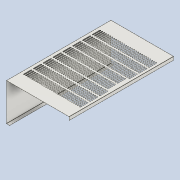
# Autodesk Inventor part: Tapa_superior_sup_ch
Saved by Autodesk Inventor 2021 (Build 250183000, 183)
## iProperties
Created: 2021-05-16
Part Number: Tapa_superior_sup_ch
Material: Acero AISI 1006 85 LC
Document SubType Name: Chapa
Designer: Admin
Density: 7.872 g/cm^3
Sheet Metal Rule: Por defecto_mm
Appearance: Acero
Author: Admin
Autodesk Inventor part; units mm, degrees
(part 1 of 2)
ref_plane "YZ Plane" through (0, 0, 0) normal (1, 0, 0) x (0, 1, 0)
ref_plane "XZ Plane" through (0, 0, 0) normal (0, 1, 0) x (-1, 0, 0)
ref_plane "XY Plane" through (0, 0, 0) normal (0, 0, 1) x (1, 0, 0)
sketch "Boceto1" plane through (0, 0, 0) normal (0, 1, 0) x (-1, 0, 0)
  line L0 (0, 0) -> (383.48, 0)
  line L1 (383.48, 0) -> (383.48, -637.48)
  line L2 (383.48, -637.48) -> (0, -637.48)
  line L3 (0, -637.48) -> (0, 0)
  dimension "d0" = 383.48
  dimension "d1" = 637.48
  measures "d0" distance of L1.end L2.end
  measures "d1" distance of L0.end L1.end
extrude "Placa1" add sketch "Boceto1" along normal blind 0.5
sketch "Boceto2" plane through (-0.5, 0.5, -637.48) normal (1, 0, 0) x (0, -1, 0)
  line L0 (0, 637.48) -> (0, 0)
  line L1 (0, 0) -> (20, 0)
  line L2 (20, 0) -> (20, 637.48)
  line L3 (20, 637.48) -> (0, 637.48)
  constraints: 6 end point, 1 horizontal, 1 perpendicular, 1 vertical
edge flange "Pestaña1" height 20 angle 90 thickness 0.5 bend radius 0.5 thickness toward (1, 0, 0) relief tear relief width 0.5 relief depth 0.25 edges at (0, 0.5, -318.74) wall of the first edge with corners at (-0.5, 0.5, 0) (-0.5, 0.5, -637.48) (-0.5, -19.5, -637.48) (-0.5, -19.5, 0)
bend "Doblez1"
corner "Esquina1"
sketch "Boceto3" plane through (-382.98, 0.5, 0) normal (-1, 0, 0) x (0, 1, 0)
  line L0 (0, -637.48) -> (0, 0)
  line L1 (0, 0) -> (-228.48, 0)
  line L2 (-228.48, 0) -> (-228.48, -637.48)
  line L3 (-228.48, -637.48) -> (0, -637.48)
  constraints: 6 end point, 1 horizontal, 1 perpendicular, 1 vertical
edge flange "Pestaña2" height 228.48 angle 90 thickness 0.5 bend radius 0.5 thickness toward (-1, 0, 0) relief tear relief width 0.5 relief depth 0.25 edges at (-383.48, 0.5, -318.74) wall of the first edge with corners at (-382.98, 0.5, -637.48) (-382.98, 0.5, 0) (-382.98, -227.98, 0) (-382.98, -227.98, -637.48)
bend "Doblez2"
corner "Esquina2"
sketch "Boceto4" plane through (-383.48, -227.48, 0) normal (0, -1, 0) x (-1, 0, 0)
  line L0 (0, -637.48) -> (0, 0)
  line L1 (0, 0) -> (-20, 0)
  line L2 (-20, 0) -> (-20, -637.48)
  line L3 (-20, -637.48) -> (0, -637.48)
  constraints: 6 end point, 1 horizontal, 1 perpendicular, 1 vertical
edge flange "Pestaña3" height 20 angle 90 thickness 0.5 bend radius 0.5 thickness toward (0, -1, 0) relief tear relief width 0.5 relief depth 0.25 edges at (-383.48, -227.98, -318.74) wall of the first edge with corners at (-383.48, -227.48, -637.48) (-383.48, -227.48, 0) (-363.48, -227.48, 0) (-363.48, -227.48, -637.48)
bend "Doblez3"
corner "Esquina3"
sketch "Boceto5" plane through (0, 0.5, 0) normal (0, 1, 0) x (1, 0, 0)
  line L0 (0, 637.48) -> (0, 0) projected
  line L1 (0, 318.74) -> (-382.98, 318.74)
  line L2 (-382.98, 637.48) -> (-382.98, 0) projected
  line L3 (-1, 0) -> (-382.48, 0) projected
  line L4 (-382.48, 637.48) -> (-1, 637.48) projected
  line L5 (-383.48, 0) -> (-383.48, 637.48) projected
  line L6 (0, 0) -> (0, 637.48) projected
  line L7 (-31.95, 313.74) -> (-31.95, 263.74) construction
  line L8 (-35.3, 310.39) -> (-35.3, 267.09)
  line L9 (-28.6, 267.09) -> (-28.6, 310.39)
  arc A0 (-28.6, 310.39) -> (-35.3, 310.39) centre (-31.95, 310.39) ccw
  arc A1 (-35.3, 267.09) -> (-28.6, 267.09) centre (-31.95, 267.09) ccw
  line L10 (-47.5, 310.39) -> (-47.5, 267.09)
  arc A2 (-47.5, 267.09) -> (-40.8, 267.09) centre (-44.15, 267.09) ccw
  line L11 (-40.8, 267.09) -> (-40.8, 310.39)
  arc A3 (-40.8, 310.39) -> (-47.5, 310.39) centre (-44.15, 310.39) ccw
  line L12 (-59.7, 310.39) -> (-59.7, 267.09)
  arc A4 (-59.7, 267.09) -> (-53, 267.09) centre (-56.35, 267.09) ccw
  line L13 (-53, 267.09) -> (-53, 310.39)
  arc A5 (-53, 310.39) -> (-59.7, 310.39) centre (-56.35, 310.39) ccw
  line L14 (-71.9, 310.39) -> (-71.9, 267.09)
  arc A6 (-71.9, 267.09) -> (-65.2, 267.09) centre (-68.55, 267.09) ccw
  line L15 (-65.2, 267.09) -> (-65.2, 310.39)
  arc A7 (-65.2, 310.39) -> (-71.9, 310.39) centre (-68.55, 310.39) ccw
  line L16 (-84.1, 310.39) -> (-84.1, 267.09)
  arc A8 (-84.1, 267.09) -> (-77.4, 267.09) centre (-80.75, 267.09) ccw
  line L17 (-77.4, 267.09) -> (-77.4, 310.39)
  arc A9 (-77.4, 310.39) -> (-84.1, 310.39) centre (-80.75, 310.39) ccw
  line L18 (-96.3, 310.39) -> (-96.3, 267.09)
  arc A10 (-96.3, 267.09) -> (-89.6, 267.09) centre (-92.95, 267.09) ccw
  line L19 (-89.6, 267.09) -> (-89.6, 310.39)
  arc A11 (-89.6, 310.39) -> (-96.3, 310.39) centre (-92.95, 310.39) ccw
  line L20 (-108.5, 310.39) -> (-108.5, 267.09)
  arc A12 (-108.5, 267.09) -> (-101.8, 267.09) centre (-105.15, 267.09) ccw
  line L21 (-101.8, 267.09) -> (-101.8, 310.39)
  arc A13 (-101.8, 310.39) -> (-108.5, 310.39) centre (-105.15, 310.39) ccw
  line L22 (-120.7, 310.39) -> (-120.7, 267.09)
  arc A14 (-120.7, 267.09) -> (-114, 267.09) centre (-117.35, 267.09) ccw
  line L23 (-114, 267.09) -> (-114, 310.39)
  arc A15 (-114, 310.39) -> (-120.7, 310.39) centre (-117.35, 310.39) ccw
  line L24 (-132.9, 310.39) -> (-132.9, 267.09)
  arc A16 (-132.9, 267.09) -> (-126.2, 267.09) centre (-129.55, 267.09) ccw
  line L25 (-126.2, 267.09) -> (-126.2, 310.39)
  arc A17 (-126.2, 310.39) -> (-132.9, 310.39) centre (-129.55, 310.39) ccw
  line L26 (-145.1, 310.39) -> (-145.1, 267.09)
  arc A18 (-145.1, 267.09) -> (-138.4, 267.09) centre (-141.75, 267.09) ccw
  line L27 (-138.4, 267.09) -> (-138.4, 310.39)
  arc A19 (-138.4, 310.39) -> (-145.1, 310.39) centre (-141.75, 310.39) ccw
  line L28 (-157.3, 310.39) -> (-157.3, 267.09)
  arc A20 (-157.3, 267.09) -> (-150.6, 267.09) centre (-153.95, 267.09) ccw
  line L29 (-150.6, 267.09) -> (-150.6, 310.39)
  arc A21 (-150.6, 310.39) -> (-157.3, 310.39) centre (-153.95, 310.39) ccw
  line L30 (-169.5, 310.39) -> (-169.5, 267.09)
  arc A22 (-169.5, 267.09) -> (-162.8, 267.09) centre (-166.15, 267.09) ccw
  line L31 (-162.8, 267.09) -> (-162.8, 310.39)
  arc A23 (-162.8, 310.39) -> (-169.5, 310.39) centre (-166.15, 310.39) ccw
  line L32 (-181.7, 310.39) -> (-181.7, 267.09)
  arc A24 (-181.7, 267.09) -> (-175, 267.09) centre (-178.35, 267.09) ccw
  line L33 (-175, 267.09) -> (-175, 310.39)
  arc A25 (-175, 310.39) -> (-181.7, 310.39) centre (-178.35, 310.39) ccw
  line L34 (-193.9, 310.39) -> (-193.9, 267.09)
  arc A26 (-193.9, 267.09) -> (-187.2, 267.09) centre (-190.55, 267.09) ccw
  line L35 (-187.2, 267.09) -> (-187.2, 310.39)
  arc A27 (-187.2, 310.39) -> (-193.9, 310.39) centre (-190.55, 310.39) ccw
  line L36 (-206.1, 310.39) -> (-206.1, 267.09)
  arc A28 (-206.1, 267.09) -> (-199.4, 267.09) centre (-202.75, 267.09) ccw
  line L37 (-199.4, 267.09) -> (-199.4, 310.39)
  arc A29 (-199.4, 310.39) -> (-206.1, 310.39) centre (-202.75, 310.39) ccw
  line L38 (-218.3, 310.39) -> (-218.3, 267.09)
  arc A30 (-218.3, 267.09) -> (-211.6, 267.09) centre (-214.95, 267.09) ccw
  line L39 (-211.6, 267.09) -> (-211.6, 310.39)
  arc A31 (-211.6, 310.39) -> (-218.3, 310.39) centre (-214.95, 310.39) ccw
  line L40 (-230.5, 310.39) -> (-230.5, 267.09)
  arc A32 (-230.5, 267.09) -> (-223.8, 267.09) centre (-227.15, 267.09) ccw
  line L41 (-223.8, 267.09) -> (-223.8, 310.39)
  arc A33 (-223.8, 310.39) -> (-230.5, 310.39) centre (-227.15, 310.39) ccw
  line L42 (-242.7, 310.39) -> (-242.7, 267.09)
  arc A34 (-242.7, 267.09) -> (-236, 267.09) centre (-239.35, 267.09) ccw
  line L43 (-236, 267.09) -> (-236, 310.39)
  arc A35 (-236, 310.39) -> (-242.7, 310.39) centre (-239.35, 310.39) ccw
  line L44 (-254.9, 310.39) -> (-254.9, 267.09)
  arc A36 (-254.9, 267.09) -> (-248.2, 267.09) centre (-251.55, 267.09) ccw
  line L45 (-248.2, 267.09) -> (-248.2, 310.39)
  arc A37 (-248.2, 310.39) -> (-254.9, 310.39) centre (-251.55, 310.39) ccw
  line L46 (-267.1, 310.39) -> (-267.1, 267.09)
  arc A38 (-267.1, 267.09) -> (-260.4, 267.09) centre (-263.75, 267.09) ccw
  line L47 (-260.4, 267.09) -> (-260.4, 310.39)
  arc A39 (-260.4, 310.39) -> (-267.1, 310.39) centre (-263.75, 310.39) ccw
  line L48 (-279.3, 310.39) -> (-279.3, 267.09)
  arc A40 (-279.3, 267.09) -> (-272.6, 267.09) centre (-275.95, 267.09) ccw
  line L49 (-272.6, 267.09) -> (-272.6, 310.39)
  arc A41 (-272.6, 310.39) -> (-279.3, 310.39) centre (-275.95, 310.39) ccw
  line L50 (-291.5, 310.39) -> (-291.5, 267.09)
  arc A42 (-291.5, 267.09) -> (-284.8, 267.09) centre (-288.15, 267.09) ccw
  line L51 (-284.8, 267.09) -> (-284.8, 310.39)
  arc A43 (-284.8, 310.39) -> (-291.5, 310.39) centre (-288.15, 310.39) ccw
  line L52 (-303.7, 310.39) -> (-303.7, 267.09)
  arc A44 (-303.7, 267.09) -> (-297, 267.09) centre (-300.35, 267.09) ccw
  line L53 (-297, 267.09) -> (-297, 310.39)
  arc A45 (-297, 310.39) -> (-303.7, 310.39) centre (-300.35, 310.39) ccw
  line L54 (-315.9, 310.39) -> (-315.9, 267.09)
  arc A46 (-315.9, 267.09) -> (-309.2, 267.09) centre (-312.55, 267.09) ccw
  line L55 (-309.2, 267.09) -> (-309.2, 310.39)
  arc A47 (-309.2, 310.39) -> (-315.9, 310.39) centre (-312.55, 310.39) ccw
  line L56 (-328.1, 310.39) -> (-328.1, 267.09)
  arc A48 (-328.1, 267.09) -> (-321.4, 267.09) centre (-324.75, 267.09) ccw
  line L57 (-321.4, 267.09) -> (-321.4, 310.39)
  arc A49 (-321.4, 310.39) -> (-328.1, 310.39) centre (-324.75, 310.39) ccw
  line L58 (-340.3, 310.39) -> (-340.3, 267.09)
  arc A50 (-340.3, 267.09) -> (-333.6, 267.09) centre (-336.95, 267.09) ccw
  line L59 (-333.6, 267.09) -> (-333.6, 310.39)
  arc A51 (-333.6, 310.39) -> (-340.3, 310.39) centre (-336.95, 310.39) ccw
  line L60 (-352.5, 310.39) -> (-352.5, 267.09)
  arc A52 (-352.5, 267.09) -> (-345.8, 267.09) centre (-349.15, 267.09) ccw
  line L61 (-345.8, 267.09) -> (-345.8, 310.39)
  arc A53 (-345.8, 310.39) -> (-352.5, 310.39) centre (-349.15, 310.39) ccw
  line L62 (-364.7, 310.39) -> (-364.7, 267.09)
  arc A54 (-364.7, 267.09) -> (-358, 267.09) centre (-361.35, 267.09) ccw
  line L63 (-358, 267.09) -> (-358, 310.39)
  arc A55 (-358, 310.39) -> (-364.7, 310.39) centre (-361.35, 310.39) ccw
  line L64 (-35.3, 250.39) -> (-35.3, 207.09)
  arc A56 (-35.3, 207.09) -> (-28.6, 207.09) centre (-31.95, 207.09) ccw
  line L65 (-28.6, 207.09) -> (-28.6, 250.39)
  arc A57 (-28.6, 250.39) -> (-35.3, 250.39) centre (-31.95, 250.39) ccw
  line L66 (-47.5, 250.39) -> (-47.5, 207.09)
  arc A58 (-47.5, 207.09) -> (-40.8, 207.09) centre (-44.15, 207.09) ccw
  line L67 (-40.8, 207.09) -> (-40.8, 250.39)
  arc A59 (-40.8, 250.39) -> (-47.5, 250.39) centre (-44.15, 250.39) ccw
  line L68 (-59.7, 250.39) -> (-59.7, 207.09)
  arc A60 (-59.7, 207.09) -> (-53, 207.09) centre (-56.35, 207.09) ccw
  line L69 (-53, 207.09) -> (-53, 250.39)
  arc A61 (-53, 250.39) -> (-59.7, 250.39) centre (-56.35, 250.39) ccw
  line L70 (-71.9, 250.39) -> (-71.9, 207.09)
  arc A62 (-71.9, 207.09) -> (-65.2, 207.09) centre (-68.55, 207.09) ccw
  line L71 (-65.2, 207.09) -> (-65.2, 250.39)
  arc A63 (-65.2, 250.39) -> (-71.9, 250.39) centre (-68.55, 250.39) ccw
  line L72 (-84.1, 250.39) -> (-84.1, 207.09)
  arc A64 (-84.1, 207.09) -> (-77.4, 207.09) centre (-80.75, 207.09) ccw
  line L73 (-77.4, 207.09) -> (-77.4, 250.39)
  arc A65 (-77.4, 250.39) -> (-84.1, 250.39) centre (-80.75, 250.39) ccw
  line L74 (-96.3, 250.39) -> (-96.3, 207.09)
  arc A66 (-96.3, 207.09) -> (-89.6, 207.09) centre (-92.95, 207.09) ccw
  line L75 (-89.6, 207.09) -> (-89.6, 250.39)
  arc A67 (-89.6, 250.39) -> (-96.3, 250.39) centre (-92.95, 250.39) ccw
  line L76 (-108.5, 250.39) -> (-108.5, 207.09)
  arc A68 (-108.5, 207.09) -> (-101.8, 207.09) centre (-105.15, 207.09) ccw
  line L77 (-101.8, 207.09) -> (-101.8, 250.39)
  arc A69 (-101.8, 250.39) -> (-108.5, 250.39) centre (-105.15, 250.39) ccw
  line L78 (-120.7, 250.39) -> (-120.7, 207.09)
  arc A70 (-120.7, 207.09) -> (-114, 207.09) centre (-117.35, 207.09) ccw
  line L79 (-114, 207.09) -> (-114, 250.39)
  arc A71 (-114, 250.39) -> (-120.7, 250.39) centre (-117.35, 250.39) ccw
  line L80 (-132.9, 250.39) -> (-132.9, 207.09)
  arc A72 (-132.9, 207.09) -> (-126.2, 207.09) centre (-129.55, 207.09) ccw
  line L81 (-126.2, 207.09) -> (-126.2, 250.39)
  arc A73 (-126.2, 250.39) -> (-132.9, 250.39) centre (-129.55, 250.39) ccw
  line L82 (-145.1, 250.39) -> (-145.1, 207.09)
  arc A74 (-145.1, 207.09) -> (-138.4, 207.09) centre (-141.75, 207.09) ccw
  line L83 (-138.4, 207.09) -> (-138.4, 250.39)
  arc A75 (-138.4, 250.39) -> (-145.1, 250.39) centre (-141.75, 250.39) ccw
  line L84 (-157.3, 250.39) -> (-157.3, 207.09)
  arc A76 (-157.3, 207.09) -> (-150.6, 207.09) centre (-153.95, 207.09) ccw
  line L85 (-150.6, 207.09) -> (-150.6, 250.39)
  arc A77 (-150.6, 250.39) -> (-157.3, 250.39) centre (-153.95, 250.39) ccw
  line L86 (-169.5, 250.39) -> (-169.5, 207.09)
  arc A78 (-169.5, 207.09) -> (-162.8, 207.09) centre (-166.15, 207.09) ccw
  line L87 (-162.8, 207.09) -> (-162.8, 250.39)
  arc A79 (-162.8, 250.39) -> (-169.5, 250.39) centre (-166.15, 250.39) ccw
  line L88 (-181.7, 250.39) -> (-181.7, 207.09)
  arc A80 (-181.7, 207.09) -> (-175, 207.09) centre (-178.35, 207.09) ccw
  line L89 (-175, 207.09) -> (-175, 250.39)
  arc A81 (-175, 250.39) -> (-181.7, 250.39) centre (-178.35, 250.39) ccw
  line L90 (-193.9, 250.39) -> (-193.9, 207.09)
  arc A82 (-193.9, 207.09) -> (-187.2, 207.09) centre (-190.55, 207.09) ccw
  line L91 (-187.2, 207.09) -> (-187.2, 250.39)
  arc A83 (-187.2, 250.39) -> (-193.9, 250.39) centre (-190.55, 250.39) ccw
  line L92 (-206.1, 250.39) -> (-206.1, 207.09)
  arc A84 (-206.1, 207.09) -> (-199.4, 207.09) centre (-202.75, 207.09) ccw
  line L93 (-199.4, 207.09) -> (-199.4, 250.39)
  arc A85 (-199.4, 250.39) -> (-206.1, 250.39) centre (-202.75, 250.39) ccw
  line L94 (-218.3, 250.39) -> (-218.3, 207.09)
  arc A86 (-218.3, 207.09) -> (-211.6, 207.09) centre (-214.95, 207.09) ccw
  line L95 (-211.6, 207.09) -> (-211.6, 250.39)
  arc A87 (-211.6, 250.39) -> (-218.3, 250.39) centre (-214.95, 250.39) ccw
  line L96 (-230.5, 250.39) -> (-230.5, 207.09)
  arc A88 (-230.5, 207.09) -> (-223.8, 207.09) centre (-227.15, 207.09) ccw
  line L97 (-223.8, 207.09) -> (-223.8, 250.39)
  arc A89 (-223.8, 250.39) -> (-230.5, 250.39) centre (-227.15, 250.39) ccw
  line L98 (-242.7, 250.39) -> (-242.7, 207.09)
  arc A90 (-242.7, 207.09) -> (-236, 207.09) centre (-239.35, 207.09) ccw
  line L99 (-236, 207.09) -> (-236, 250.39)
  arc A91 (-236, 250.39) -> (-242.7, 250.39) centre (-239.35, 250.39) ccw
  line L100 (-254.9, 250.39) -> (-254.9, 207.09)
  arc A92 (-254.9, 207.09) -> (-248.2, 207.09) centre (-251.55, 207.09) ccw
  line L101 (-248.2, 207.09) -> (-248.2, 250.39)
  arc A93 (-248.2, 250.39) -> (-254.9, 250.39) centre (-251.55, 250.39) ccw
  line L102 (-267.1, 250.39) -> (-267.1, 207.09)
  arc A94 (-267.1, 207.09) -> (-260.4, 207.09) centre (-263.75, 207.09) ccw
  line L103 (-260.4, 207.09) -> (-260.4, 250.39)
  arc A95 (-260.4, 250.39) -> (-267.1, 250.39) centre (-263.75, 250.39) ccw
  line L104 (-279.3, 250.39) -> (-279.3, 207.09)
  arc A96 (-279.3, 207.09) -> (-272.6, 207.09) centre (-275.95, 207.09) ccw
  line L105 (-272.6, 207.09) -> (-272.6, 250.39)
  arc A97 (-272.6, 250.39) -> (-279.3, 250.39) centre (-275.95, 250.39) ccw
  line L106 (-291.5, 250.39) -> (-291.5, 207.09)
  arc A98 (-291.5, 207.09) -> (-284.8, 207.09) centre (-288.15, 207.09) ccw
  line L107 (-284.8, 207.09) -> (-284.8, 250.39)
  arc A99 (-284.8, 250.39) -> (-291.5, 250.39) centre (-288.15, 250.39) ccw
  line L108 (-303.7, 250.39) -> (-303.7, 207.09)
  arc A100 (-303.7, 207.09) -> (-297, 207.09) centre (-300.35, 207.09) ccw
  line L109 (-297, 207.09) -> (-297, 250.39)
  arc A101 (-297, 250.39) -> (-303.7, 250.39) centre (-300.35, 250.39) ccw
  line L110 (-315.9, 250.39) -> (-315.9, 207.09)
  arc A102 (-315.9, 207.09) -> (-309.2, 207.09) centre (-312.55, 207.09) ccw
  line L111 (-309.2, 207.09) -> (-309.2, 250.39)
  arc A103 (-309.2, 250.39) -> (-315.9, 250.39) centre (-312.55, 250.39) ccw
  line L112 (-328.1, 250.39) -> (-328.1, 207.09)
  arc A104 (-328.1, 207.09) -> (-321.4, 207.09) centre (-324.75, 207.09) ccw
  line L113 (-321.4, 207.09) -> (-321.4, 250.39)
  arc A105 (-321.4, 250.39) -> (-328.1, 250.39) centre (-324.75, 250.39) ccw
  line L114 (-340.3, 250.39) -> (-340.3, 207.09)
  arc A106 (-340.3, 207.09) -> (-333.6, 207.09) centre (-336.95, 207.09) ccw
  line L115 (-333.6, 207.09) -> (-333.6, 250.39)
  arc A107 (-333.6, 250.39) -> (-340.3, 250.39) centre (-336.95, 250.39) ccw
  line L116 (-352.5, 250.39) -> (-352.5, 207.09)
  arc A108 (-352.5, 207.09) -> (-345.8, 207.09) centre (-349.15, 207.09) ccw
  line L117 (-345.8, 207.09) -> (-345.8, 250.39)
  arc A109 (-345.8, 250.39) -> (-352.5, 250.39) centre (-349.15, 250.39) ccw
  line L118 (-364.7, 250.39) -> (-364.7, 207.09)
  arc A110 (-364.7, 207.09) -> (-358, 207.09) centre (-361.35, 207.09) ccw
  line L119 (-358, 207.09) -> (-358, 250.39)
  arc A111 (-358, 250.39) -> (-364.7, 250.39) centre (-361.35, 250.39) ccw
  line L120 (-35.3, 190.39) -> (-35.3, 147.09)
  arc A112 (-35.3, 147.09) -> (-28.6, 147.09) centre (-31.95, 147.09) ccw
  line L121 (-28.6, 147.09) -> (-28.6, 190.39)
  arc A113 (-28.6, 190.39) -> (-35.3, 190.39) centre (-31.95, 190.39) ccw
  line L122 (-47.5, 190.39) -> (-47.5, 147.09)
  arc A114 (-47.5, 147.09) -> (-40.8, 147.09) centre (-44.15, 147.09) ccw
  line L123 (-40.8, 147.09) -> (-40.8, 190.39)
  arc A115 (-40.8, 190.39) -> (-47.5, 190.39) centre (-44.15, 190.39) ccw
  line L124 (-59.7, 190.39) -> (-59.7, 147.09)
  arc A116 (-59.7, 147.09) -> (-53, 147.09) centre (-56.35, 147.09) ccw
  line L125 (-53, 147.09) -> (-53, 190.39)
  arc A117 (-53, 190.39) -> (-59.7, 190.39) centre (-56.35, 190.39) ccw
  line L126 (-71.9, 190.39) -> (-71.9, 147.09)
  arc A118 (-71.9, 147.09) -> (-65.2, 147.09) centre (-68.55, 147.09) ccw
  line L127 (-65.2, 147.09) -> (-65.2, 190.39)
  arc A119 (-65.2, 190.39) -> (-71.9, 190.39) centre (-68.55, 190.39) ccw
  line L128 (-84.1, 190.39) -> (-84.1, 147.09)
  arc A120 (-84.1, 147.09) -> (-77.4, 147.09) centre (-80.75, 147.09) ccw
  line L129 (-77.4, 147.09) -> (-77.4, 190.39)
  arc A121 (-77.4, 190.39) -> (-84.1, 190.39) centre (-80.75, 190.39) ccw
  line L130 (-96.3, 190.39) -> (-96.3, 147.09)
  arc A122 (-96.3, 147.09) -> (-89.6, 147.09) centre (-92.95, 147.09) ccw
  line L131 (-89.6, 147.09) -> (-89.6, 190.39)
  arc A123 (-89.6, 190.39) -> (-96.3, 190.39) centre (-92.95, 190.39) ccw
  line L132 (-108.5, 190.39) -> (-108.5, 147.09)
  arc A124 (-108.5, 147.09) -> (-101.8, 147.09) centre (-105.15, 147.09) ccw
  line L133 (-101.8, 147.09) -> (-101.8, 190.39)
  arc A125 (-101.8, 190.39) -> (-108.5, 190.39) centre (-105.15, 190.39) ccw
  line L134 (-120.7, 190.39) -> (-120.7, 147.09)
  arc A126 (-120.7, 147.09) -> (-114, 147.09) centre (-117.35, 147.09) ccw
  line L135 (-114, 147.09) -> (-114, 190.39)
  arc A127 (-114, 190.39) -> (-120.7, 190.39) centre (-117.35, 190.39) ccw
  line L136 (-132.9, 190.39) -> (-132.9, 147.09)
  arc A128 (-132.9, 147.09) -> (-126.2, 147.09) centre (-129.55, 147.09) ccw
  line L137 (-126.2, 147.09) -> (-126.2, 190.39)
  arc A129 (-126.2, 190.39) -> (-132.9, 190.39) centre (-129.55, 190.39) ccw
  line L138 (-145.1, 190.39) -> (-145.1, 147.09)
  arc A130 (-145.1, 147.09) -> (-138.4, 147.09) centre (-141.75, 147.09) ccw
  line L139 (-138.4, 147.09) -> (-138.4, 190.39)
  arc A131 (-138.4, 190.39) -> (-145.1, 190.39) centre (-141.75, 190.39) ccw
  line L140 (-157.3, 190.39) -> (-157.3, 147.09)
  arc A132 (-157.3, 147.09) -> (-150.6, 147.09) centre (-153.95, 147.09) ccw
  line L141 (-150.6, 147.09) -> (-150.6, 190.39)
  arc A133 (-150.6, 190.39) -> (-157.3, 190.39) centre (-153.95, 190.39) ccw
  line L142 (-169.5, 190.39) -> (-169.5, 147.09)
  arc A134 (-169.5, 147.09) -> (-162.8, 147.09) centre (-166.15, 147.09) ccw
  line L143 (-162.8, 147.09) -> (-162.8, 190.39)
  arc A135 (-162.8, 190.39) -> (-169.5, 190.39) centre (-166.15, 190.39) ccw
  line L144 (-181.7, 190.39) -> (-181.7, 147.09)
  arc A136 (-181.7, 147.09) -> (-175, 147.09) centre (-178.35, 147.09) ccw
  line L145 (-175, 147.09) -> (-175, 190.39)
  arc A137 (-175, 190.39) -> (-181.7, 190.39) centre (-178.35, 190.39) ccw
  line L146 (-193.9, 190.39) -> (-193.9, 147.09)
  arc A138 (-193.9, 147.09) -> (-187.2, 147.09) centre (-190.55, 147.09) ccw
  line L147 (-187.2, 147.09) -> (-187.2, 190.39)
  arc A139 (-187.2, 190.39) -> (-193.9, 190.39) centre (-190.55, 190.39) ccw
  line L148 (-206.1, 190.39) -> (-206.1, 147.09)
  arc A140 (-206.1, 147.09) -> (-199.4, 147.09) centre (-202.75, 147.09) ccw
  line L149 (-199.4, 147.09) -> (-199.4, 190.39)
  arc A141 (-199.4, 190.39) -> (-206.1, 190.39) centre (-202.75, 190.39) ccw
  line L150 (-218.3, 190.39) -> (-218.3, 147.09)
  arc A142 (-218.3, 147.09) -> (-211.6, 147.09) centre (-214.95, 147.09) ccw
  line L151 (-211.6, 147.09) -> (-211.6, 190.39)
  arc A143 (-211.6, 190.39) -> (-218.3, 190.39) centre (-214.95, 190.39) ccw
  line L152 (-230.5, 190.39) -> (-230.5, 147.09)
  arc A144 (-230.5, 147.09) -> (-223.8, 147.09) centre (-227.15, 147.09) ccw
  line L153 (-223.8, 147.09) -> (-223.8, 190.39)
  arc A145 (-223.8, 190.39) -> (-230.5, 190.39) centre (-227.15, 190.39) ccw
  line L154 (-242.7, 190.39) -> (-242.7, 147.09)
  arc A146 (-242.7, 147.09) -> (-236, 147.09) centre (-239.35, 147.09) ccw
  line L155 (-236, 147.09) -> (-236, 190.39)
  arc A147 (-236, 190.39) -> (-242.7, 190.39) centre (-239.35, 190.39) ccw
  line L156 (-254.9, 190.39) -> (-254.9, 147.09)
  arc A148 (-254.9, 147.09) -> (-248.2, 147.09) centre (-251.55, 147.09) ccw
  line L157 (-248.2, 147.09) -> (-248.2, 190.39)
  arc A149 (-248.2, 190.39) -> (-254.9, 190.39) centre (-251.55, 190.39) ccw
  line L158 (-267.1, 190.39) -> (-267.1, 147.09)
  arc A150 (-267.1, 147.09) -> (-260.4, 147.09) centre (-263.75, 147.09) ccw
  line L159 (-260.4, 147.09) -> (-260.4, 190.39)
  arc A151 (-260.4, 190.39) -> (-267.1, 190.39) centre (-263.75, 190.39) ccw
  line L160 (-279.3, 190.39) -> (-279.3, 147.09)
  arc A152 (-279.3, 147.09) -> (-272.6, 147.09) centre (-275.95, 147.09) ccw
  line L161 (-272.6, 147.09) -> (-272.6, 190.39)
  arc A153 (-272.6, 190.39) -> (-279.3, 190.39) centre (-275.95, 190.39) ccw
  line L162 (-291.5, 190.39) -> (-291.5, 147.09)
  arc A154 (-291.5, 147.09) -> (-284.8, 147.09) centre (-288.15, 147.09) ccw
  line L163 (-284.8, 147.09) -> (-284.8, 190.39)
  arc A155 (-284.8, 190.39) -> (-291.5, 190.39) centre (-288.15, 190.39) ccw
  line L164 (-303.7, 190.39) -> (-303.7, 147.09)
  arc A156 (-303.7, 147.09) -> (-297, 147.09) centre (-300.35, 147.09) ccw
  line L165 (-297, 147.09) -> (-297, 190.39)
  arc A157 (-297, 190.39) -> (-303.7, 190.39) centre (-300.35, 190.39) ccw
  line L166 (-315.9, 190.39) -> (-315.9, 147.09)
  arc A158 (-315.9, 147.09) -> (-309.2, 147.09) centre (-312.55, 147.09) ccw
  line L167 (-309.2, 147.09) -> (-309.2, 190.39)
  arc A159 (-309.2, 190.39) -> (-315.9, 190.39) centre (-312.55, 190.39) ccw
  line L168 (-328.1, 190.39) -> (-328.1, 147.09)
  arc A160 (-328.1, 147.09) -> (-321.4, 147.09) centre (-324.75, 147.09) ccw
  line L169 (-321.4, 147.09) -> (-321.4, 190.39)
  arc A161 (-321.4, 190.39) -> (-328.1, 190.39) centre (-324.75, 190.39) ccw
  line L170 (-340.3, 190.39) -> (-340.3, 147.09)
  arc A162 (-340.3, 147.09) -> (-333.6, 147.09) centre (-336.95, 147.09) ccw
  line L171 (-333.6, 147.09) -> (-333.6, 190.39)
  arc A163 (-333.6, 190.39) -> (-340.3, 190.39) centre (-336.95, 190.39) ccw
  line L172 (-352.5, 190.39) -> (-352.5, 147.09)
  arc A164 (-352.5, 147.09) -> (-345.8, 147.09) centre (-349.15, 147.09) ccw
  line L173 (-345.8, 147.09) -> (-345.8, 190.39)
  arc A165 (-345.8, 190.39) -> (-352.5, 190.39) centre (-349.15, 190.39) ccw
  line L174 (-364.7, 190.39) -> (-364.7, 147.09)
  arc A166 (-364.7, 147.09) -> (-358, 147.09) centre (-361.35, 147.09) ccw
  line L175 (-358, 147.09) -> (-358, 190.39)
  arc A167 (-358, 190.39) -> (-364.7, 190.39) centre (-361.35, 190.39) ccw
  line L176 (-35.3, 130.39) -> (-35.3, 87.09)
  arc A168 (-35.3, 87.09) -> (-28.6, 87.09) centre (-31.95, 87.09) ccw
  line L177 (-28.6, 87.09) -> (-28.6, 130.39)
  arc A169 (-28.6, 130.39) -> (-35.3, 130.39) centre (-31.95, 130.39) ccw
  line L178 (-47.5, 130.39) -> (-47.5, 87.09)
  arc A170 (-47.5, 87.09) -> (-40.8, 87.09) centre (-44.15, 87.09) ccw
  line L179 (-40.8, 87.09) -> (-40.8, 130.39)
  arc A171 (-40.8, 130.39) -> (-47.5, 130.39) centre (-44.15, 130.39) ccw
  line L180 (-59.7, 130.39) -> (-59.7, 87.09)
  arc A172 (-59.7, 87.09) -> (-53, 87.09) centre (-56.35, 87.09) ccw
  line L181 (-53, 87.09) -> (-53, 130.39)
  arc A173 (-53, 130.39) -> (-59.7, 130.39) centre (-56.35, 130.39) ccw
  line L182 (-71.9, 130.39) -> (-71.9, 87.09)
  arc A174 (-71.9, 87.09) -> (-65.2, 87.09) centre (-68.55, 87.09) ccw
  line L183 (-65.2, 87.09) -> (-65.2, 130.39)
  arc A175 (-65.2, 130.39) -> (-71.9, 130.39) centre (-68.55, 130.39) ccw
  line L184 (-84.1, 130.39) -> (-84.1, 87.09)
  arc A176 (-84.1, 87.09) -> (-77.4, 87.09) centre (-80.75, 87.09) ccw
  line L185 (-77.4, 87.09) -> (-77.4, 130.39)
  arc A177 (-77.4, 130.39) -> (-84.1, 130.39) centre (-80.75, 130.39) ccw
  line L186 (-96.3, 130.39) -> (-96.3, 87.09)
  arc A178 (-96.3, 87.09) -> (-89.6, 87.09) centre (-92.95, 87.09) ccw
  line L187 (-89.6, 87.09) -> (-89.6, 130.39)
  arc A179 (-89.6, 130.39) -> (-96.3, 130.39) centre (-92.95, 130.39) ccw
  line L188 (-108.5, 130.39) -> (-108.5, 87.09)
  arc A180 (-108.5, 87.09) -> (-101.8, 87.09) centre (-105.15, 87.09) ccw
  line L189 (-101.8, 87.09) -> (-101.8, 130.39)
  arc A181 (-101.8, 130.39) -> (-108.5, 130.39) centre (-105.15, 130.39) ccw
  line L190 (-120.7, 130.39) -> (-120.7, 87.09)
  arc A182 (-120.7, 87.09) -> (-114, 87.09) centre (-117.35, 87.09) ccw
  line L191 (-114, 87.09) -> (-114, 130.39)
  arc A183 (-114, 130.39) -> (-120.7, 130.39) centre (-117.35, 130.39) ccw
  line L192 (-132.9, 130.39) -> (-132.9, 87.09)
  arc A184 (-132.9, 87.09) -> (-126.2, 87.09) centre (-129.55, 87.09) ccw
  line L193 (-126.2, 87.09) -> (-126.2, 130.39)
  arc A185 (-126.2, 130.39) -> (-132.9, 130.39) centre (-129.55, 130.39) ccw
  line L194 (-145.1, 130.39) -> (-145.1, 87.09)
  arc A186 (-145.1, 87.09) -> (-138.4, 87.09) centre (-141.75, 87.09) ccw
  line L195 (-138.4, 87.09) -> (-138.4, 130.39)
  arc A187 (-138.4, 130.39) -> (-145.1, 130.39) centre (-141.75, 130.39) ccw
  line L196 (-157.3, 130.39) -> (-157.3, 87.09)
  arc A188 (-157.3, 87.09) -> (-150.6, 87.09) centre (-153.95, 87.09) ccw
  line L197 (-150.6, 87.09) -> (-150.6, 130.39)
  arc A189 (-150.6, 130.39) -> (-157.3, 130.39) centre (-153.95, 130.39) ccw
  line L198 (-169.5, 130.39) -> (-169.5, 87.09)
  arc A190 (-169.5, 87.09) -> (-162.8, 87.09) centre (-166.15, 87.09) ccw
  line L199 (-162.8, 87.09) -> (-162.8, 130.39)
  arc A191 (-162.8, 130.39) -> (-169.5, 130.39) centre (-166.15, 130.39) ccw
  line L200 (-181.7, 130.39) -> (-181.7, 87.09)
  arc A192 (-181.7, 87.09) -> (-175, 87.09) centre (-178.35, 87.09) ccw
  line L201 (-175, 87.09) -> (-175, 130.39)
  arc A193 (-175, 130.39) -> (-181.7, 130.39) centre (-178.35, 130.39) ccw
  line L202 (-193.9, 130.39) -> (-193.9, 87.09)
  arc A194 (-193.9, 87.09) -> (-187.2, 87.09) centre (-190.55, 87.09) ccw
  line L203 (-187.2, 87.09) -> (-187.2, 130.39)
  arc A195 (-187.2, 130.39) -> (-193.9, 130.39) centre (-190.55, 130.39) ccw
  line L204 (-206.1, 130.39) -> (-206.1, 87.09)
  arc A196 (-206.1, 87.09) -> (-199.4, 87.09) centre (-202.75, 87.09) ccw
  line L205 (-199.4, 87.09) -> (-199.4, 130.39)
  arc A197 (-199.4, 130.39) -> (-206.1, 130.39) centre (-202.75, 130.39) ccw
  line L206 (-218.3, 130.39) -> (-218.3, 87.09)
  arc A198 (-218.3, 87.09) -> (-211.6, 87.09) centre (-214.95, 87.09) ccw
  line L207 (-211.6, 87.09) -> (-211.6, 130.39)
  arc A199 (-211.6, 130.39) -> (-218.3, 130.39) centre (-214.95, 130.39) ccw
  line L208 (-230.5, 130.39) -> (-230.5, 87.09)
  arc A200 (-230.5, 87.09) -> (-223.8, 87.09) centre (-227.15, 87.09) ccw
  line L209 (-223.8, 87.09) -> (-223.8, 130.39)
  arc A201 (-223.8, 130.39) -> (-230.5, 130.39) centre (-227.15, 130.39) ccw
  line L210 (-242.7, 130.39) -> (-242.7, 87.09)
  arc A202 (-242.7, 87.09) -> (-236, 87.09) centre (-239.35, 87.09) ccw
  line L211 (-236, 87.09) -> (-236, 130.39)
  arc A203 (-236, 130.39) -> (-242.7, 130.39) centre (-239.35, 130.39) ccw
  line L212 (-254.9, 130.39) -> (-254.9, 87.09)
  arc A204 (-254.9, 87.09) -> (-248.2, 87.09) centre (-251.55, 87.09) ccw
  line L213 (-248.2, 87.09) -> (-248.2, 130.39)
  arc A205 (-248.2, 130.39) -> (-254.9, 130.39) centre (-251.55, 130.39) ccw
  line L214 (-267.1, 130.39) -> (-267.1, 87.09)
  arc A206 (-267.1, 87.09) -> (-260.4, 87.09) centre (-263.75, 87.09) ccw
  line L215 (-260.4, 87.09) -> (-260.4, 130.39)
  arc A207 (-260.4, 130.39) -> (-267.1, 130.39) centre (-263.75, 130.39) ccw
  line L216 (-279.3, 130.39) -> (-279.3, 87.09)
  arc A208 (-279.3, 87.09) -> (-272.6, 87.09) centre (-275.95, 87.09) ccw
  line L217 (-272.6, 87.09) -> (-272.6, 130.39)
  arc A209 (-272.6, 130.39) -> (-279.3, 130.39) centre (-275.95, 130.39) ccw
  line L218 (-291.5, 130.39) -> (-291.5, 87.09)
  arc A210 (-291.5, 87.09) -> (-284.8, 87.09) centre (-288.15, 87.09) ccw
  line L219 (-284.8, 87.09) -> (-284.8, 130.39)
  arc A211 (-284.8, 130.39) -> (-291.5, 130.39) centre (-288.15, 130.39) ccw
  line L220 (-303.7, 130.39) -> (-303.7, 87.09)
  arc A212 (-303.7, 87.09) -> (-297, 87.09) centre (-300.35, 87.09) ccw
  line L221 (-297, 87.09) -> (-297, 130.39)
  arc A213 (-297, 130.39) -> (-303.7, 130.39) centre (-300.35, 130.39) ccw
  line L222 (-315.9, 130.39) -> (-315.9, 87.09)
  arc A214 (-315.9, 87.09) -> (-309.2, 87.09) centre (-312.55, 87.09) ccw
  line L223 (-309.2, 87.09) -> (-309.2, 130.39)
  arc A215 (-309.2, 130.39) -> (-315.9, 130.39) centre (-312.55, 130.39) ccw
  line L224 (-328.1, 130.39) -> (-328.1, 87.09)
  arc A216 (-328.1, 87.09) -> (-321.4, 87.09) centre (-324.75, 87.09) ccw
  line L225 (-321.4, 87.09) -> (-321.4, 130.39)
  arc A217 (-321.4, 130.39) -> (-328.1, 130.39) centre (-324.75, 130.39) ccw
  line L226 (-340.3, 130.39) -> (-340.3, 87.09)
  arc A218 (-340.3, 87.09) -> (-333.6, 87.09) centre (-336.95, 87.09) ccw
  line L227 (-333.6, 87.09) -> (-333.6, 130.39)
  arc A219 (-333.6, 130.39) -> (-340.3, 130.39) centre (-336.95, 130.39) ccw
  line L228 (-352.5, 130.39) -> (-352.5, 87.09)
  arc A220 (-352.5, 87.09) -> (-345.8, 87.09) centre (-349.15, 87.09) ccw
  line L229 (-345.8, 87.09) -> (-345.8, 130.39)
  arc A221 (-345.8, 130.39) -> (-352.5, 130.39) centre (-349.15, 130.39) ccw
  line L230 (-364.7, 130.39) -> (-364.7, 87.09)
  arc A222 (-364.7, 87.09) -> (-358, 87.09) centre (-361.35, 87.09) ccw
  line L231 (-358, 87.09) -> (-358, 130.39)
  arc A223 (-358, 130.39) -> (-364.7, 130.39) centre (-361.35, 130.39) ccw
  line L232 (-19.75, 253.74) -> (-19.75, 203.74) construction
  line L233 (-16.4, 250.39) -> (-16.4, 207.09)
  line L234 (-23.1, 207.09) -> (-23.1, 250.39)
  arc A224 (-16.4, 250.39) -> (-23.1, 250.39) centre (-19.75, 250.39) ccw
  arc A225 (-23.1, 207.09) -> (-16.4, 207.09) centre (-19.75, 207.09) ccw
  line L235 (-23.1, 147.09) -> (-23.1, 190.39)
  arc A226 (-23.1, 147.09) -> (-16.4, 147.09) centre (-19.75, 147.09) ccw
  line L236 (-16.4, 190.39) -> (-16.4, 147.09)
  arc A227 (-16.4, 190.39) -> (-23.1, 190.39) centre (-19.75, 190.39) ccw
  line L237 (-23.1, 87.09) -> (-23.1, 130.39)
  arc A228 (-23.1, 87.09) -> (-16.4, 87.09) centre (-19.75, 87.09) ccw
  line L238 (-16.4, 130.39) -> (-16.4, 87.09)
  arc A229 (-16.4, 130.39) -> (-23.1, 130.39) centre (-19.75, 130.39) ccw
  line L239 (-31.95, 323.74) -> (-31.95, 373.74) construction
  line L240 (-35.3, 327.09) -> (-35.3, 370.39)
  line L241 (-28.6, 370.39) -> (-28.6, 327.09)
  arc A230 (-35.3, 327.09) -> (-28.6, 327.09) centre (-31.95, 327.09) ccw
  arc A231 (-28.6, 370.39) -> (-35.3, 370.39) centre (-31.95, 370.39) ccw
  line L242 (-47.5, 327.09) -> (-47.5, 370.39)
  arc A232 (-40.8, 370.39) -> (-47.5, 370.39) centre (-44.15, 370.39) ccw
  line L243 (-40.8, 370.39) -> (-40.8, 327.09)
  arc A233 (-47.5, 327.09) -> (-40.8, 327.09) centre (-44.15, 327.09) ccw
  line L244 (-59.7, 327.09) -> (-59.7, 370.39)
  arc A234 (-53, 370.39) -> (-59.7, 370.39) centre (-56.35, 370.39) ccw
  line L245 (-53, 370.39) -> (-53, 327.09)
  arc A235 (-59.7, 327.09) -> (-53, 327.09) centre (-56.35, 327.09) ccw
  line L246 (-71.9, 327.09) -> (-71.9, 370.39)
  arc A236 (-65.2, 370.39) -> (-71.9, 370.39) centre (-68.55, 370.39) ccw
  line L247 (-65.2, 370.39) -> (-65.2, 327.09)
  arc A237 (-71.9, 327.09) -> (-65.2, 327.09) centre (-68.55, 327.09) ccw
  line L248 (-84.1, 327.09) -> (-84.1, 370.39)
  arc A238 (-77.4, 370.39) -> (-84.1, 370.39) centre (-80.75, 370.39) ccw
  line L249 (-77.4, 370.39) -> (-77.4, 327.09)
  arc A239 (-84.1, 327.09) -> (-77.4, 327.09) centre (-80.75, 327.09) ccw
  line L250 (-96.3, 327.09) -> (-96.3, 370.39)
  arc A240 (-89.6, 370.39) -> (-96.3, 370.39) centre (-92.95, 370.39) ccw
  line L251 (-89.6, 370.39) -> (-89.6, 327.09)
  arc A241 (-96.3, 327.09) -> (-89.6, 327.09) centre (-92.95, 327.09) ccw
  line L252 (-108.5, 327.09) -> (-108.5, 370.39)
  arc A242 (-101.8, 370.39) -> (-108.5, 370.39) centre (-105.15, 370.39) ccw
  line L253 (-101.8, 370.39) -> (-101.8, 327.09)
  arc A243 (-108.5, 327.09) -> (-101.8, 327.09) centre (-105.15, 327.09) ccw
  line L254 (-120.7, 327.09) -> (-120.7, 370.39)
  arc A244 (-114, 370.39) -> (-120.7, 370.39) centre (-117.35, 370.39) ccw
  line L255 (-114, 370.39) -> (-114, 327.09)
  arc A245 (-120.7, 327.09) -> (-114, 327.09) centre (-117.35, 327.09) ccw
  line L256 (-132.9, 327.09) -> (-132.9, 370.39)
  arc A246 (-126.2, 370.39) -> (-132.9, 370.39) centre (-129.55, 370.39) ccw
  line L257 (-126.2, 370.39) -> (-126.2, 327.09)
  arc A247 (-132.9, 327.09) -> (-126.2, 327.09) centre (-129.55, 327.09) ccw
  line L258 (-145.1, 327.09) -> (-145.1, 370.39)
  arc A248 (-138.4, 370.39) -> (-145.1, 370.39) centre (-141.75, 370.39) ccw
  line L259 (-138.4, 370.39) -> (-138.4, 327.09)
  arc A249 (-145.1, 327.09) -> (-138.4, 327.09) centre (-141.75, 327.09) ccw
  line L260 (-157.3, 327.09) -> (-157.3, 370.39)
  arc A250 (-150.6, 370.39) -> (-157.3, 370.39) centre (-153.95, 370.39) ccw
  line L261 (-150.6, 370.39) -> (-150.6, 327.09)
  arc A251 (-157.3, 327.09) -> (-150.6, 327.09) centre (-153.95, 327.09) ccw
  line L262 (-169.5, 327.09) -> (-169.5, 370.39)
  arc A252 (-162.8, 370.39) -> (-169.5, 370.39) centre (-166.15, 370.39) ccw
  line L263 (-162.8, 370.39) -> (-162.8, 327.09)
  arc A253 (-169.5, 327.09) -> (-162.8, 327.09) centre (-166.15, 327.09) ccw
  line L264 (-181.7, 327.09) -> (-181.7, 370.39)
  arc A254 (-175, 370.39) -> (-181.7, 370.39) centre (-178.35, 370.39) ccw
  line L265 (-175, 370.39) -> (-175, 327.09)
  arc A255 (-181.7, 327.09) -> (-175, 327.09) centre (-178.35, 327.09) ccw
  line L266 (-193.9, 327.09) -> (-193.9, 370.39)
  arc A256 (-187.2, 370.39) -> (-193.9, 370.39) centre (-190.55, 370.39) ccw
  line L267 (-187.2, 370.39) -> (-187.2, 327.09)
  arc A257 (-193.9, 327.09) -> (-187.2, 327.09) centre (-190.55, 327.09) ccw
  line L268 (-206.1, 327.09) -> (-206.1, 370.39)
  arc A258 (-199.4, 370.39) -> (-206.1, 370.39) centre (-202.75, 370.39) ccw
  line L269 (-199.4, 370.39) -> (-199.4, 327.09)
  arc A259 (-206.1, 327.09) -> (-199.4, 327.09) centre (-202.75, 327.09) ccw
  line L270 (-218.3, 327.09) -> (-218.3, 370.39)
  arc A260 (-211.6, 370.39) -> (-218.3, 370.39) centre (-214.95, 370.39) ccw
  line L271 (-211.6, 370.39) -> (-211.6, 327.09)
  arc A261 (-218.3, 327.09) -> (-211.6, 327.09) centre (-214.95, 327.09) ccw
  line L272 (-230.5, 327.09) -> (-230.5, 370.39)
  arc A262 (-223.8, 370.39) -> (-230.5, 370.39) centre (-227.15, 370.39) ccw
  line L273 (-223.8, 370.39) -> (-223.8, 327.09)
  arc A263 (-230.5, 327.09) -> (-223.8, 327.09) centre (-227.15, 327.09) ccw
  line L274 (-242.7, 327.09) -> (-242.7, 370.39)
  arc A264 (-236, 370.39) -> (-242.7, 370.39) centre (-239.35, 370.39) ccw
  line L275 (-236, 370.39) -> (-236, 327.09)
  arc A265 (-242.7, 327.09) -> (-236, 327.09) centre (-239.35, 327.09) ccw
  line L276 (-254.9, 327.09) -> (-254.9, 370.39)
  arc A266 (-248.2, 370.39) -> (-254.9, 370.39) centre (-251.55, 370.39) ccw
  line L277 (-248.2, 370.39) -> (-248.2, 327.09)
  arc A267 (-254.9, 327.09) -> (-248.2, 327.09) centre (-251.55, 327.09) ccw
  line L278 (-267.1, 327.09) -> (-267.1, 370.39)
  arc A268 (-260.4, 370.39) -> (-267.1, 370.39) centre (-263.75, 370.39) ccw
  line L279 (-260.4, 370.39) -> (-260.4, 327.09)
  arc A269 (-267.1, 327.09) -> (-260.4, 327.09) centre (-263.75, 327.09) ccw
  line L280 (-279.3, 327.09) -> (-279.3, 370.39)
  arc A270 (-272.6, 370.39) -> (-279.3, 370.39) centre (-275.95, 370.39) ccw
  line L281 (-272.6, 370.39) -> (-272.6, 327.09)
  arc A271 (-279.3, 327.09) -> (-272.6, 327.09) centre (-275.95, 327.09) ccw
  line L282 (-291.5, 327.09) -> (-291.5, 370.39)
  arc A272 (-284.8, 370.39) -> (-291.5, 370.39) centre (-288.15, 370.39) ccw
  line L283 (-284.8, 370.39) -> (-284.8, 327.09)
  arc A273 (-291.5, 327.09) -> (-284.8, 327.09) centre (-288.15, 327.09) ccw
  line L284 (-303.7, 327.09) -> (-303.7, 370.39)
  arc A274 (-297, 370.39) -> (-303.7, 370.39) centre (-300.35, 370.39) ccw
  line L285 (-297, 370.39) -> (-297, 327.09)
  arc A275 (-303.7, 327.09) -> (-297, 327.09) centre (-300.35, 327.09) ccw
  line L286 (-315.9, 327.09) -> (-315.9, 370.39)
  arc A276 (-309.2, 370.39) -> (-315.9, 370.39) centre (-312.55, 370.39) ccw
  line L287 (-309.2, 370.39) -> (-309.2, 327.09)
  arc A277 (-315.9, 327.09) -> (-309.2, 327.09) centre (-312.55, 327.09) ccw
  line L288 (-328.1, 327.09) -> (-328.1, 370.39)
  arc A278 (-321.4, 370.39) -> (-328.1, 370.39) centre (-324.75, 370.39) ccw
  line L289 (-321.4, 370.39) -> (-321.4, 327.09)
  arc A279 (-328.1, 327.09) -> (-321.4, 327.09) centre (-324.75, 327.09) ccw
  line L290 (-340.3, 327.09) -> (-340.3, 370.39)
  arc A280 (-333.6, 370.39) -> (-340.3, 370.39) centre (-336.95, 370.39) ccw
  line L291 (-333.6, 370.39) -> (-333.6, 327.09)
  arc A281 (-340.3, 327.09) -> (-333.6, 327.09) centre (-336.95, 327.09) ccw
  line L292 (-352.5, 327.09) -> (-352.5, 370.39)
  arc A282 (-345.8, 370.39) -> (-352.5, 370.39) centre (-349.15, 370.39) ccw
  line L293 (-345.8, 370.39) -> (-345.8, 327.09)
  arc A283 (-352.5, 327.09) -> (-345.8, 327.09) centre (-349.15, 327.09) ccw
  line L294 (-364.7, 327.09) -> (-364.7, 370.39)
  arc A284 (-358, 370.39) -> (-364.7, 370.39) centre (-361.35, 370.39) ccw
  line L295 (-358, 370.39) -> (-358, 327.09)
  arc A285 (-364.7, 327.09) -> (-358, 327.09) centre (-361.35, 327.09) ccw
  line L296 (-35.3, 387.09) -> (-35.3, 430.39)
  arc A286 (-28.6, 430.39) -> (-35.3, 430.39) centre (-31.95, 430.39) ccw
  line L297 (-28.6, 430.39) -> (-28.6, 387.09)
  arc A287 (-35.3, 387.09) -> (-28.6, 387.09) centre (-31.95, 387.09) ccw
  line L298 (-47.5, 387.09) -> (-47.5, 430.39)
  arc A288 (-40.8, 430.39) -> (-47.5, 430.39) centre (-44.15, 430.39) ccw
  line L299 (-40.8, 430.39) -> (-40.8, 387.09)
  arc A289 (-47.5, 387.09) -> (-40.8, 387.09) centre (-44.15, 387.09) ccw
  line L300 (-59.7, 387.09) -> (-59.7, 430.39)
  arc A290 (-53, 430.39) -> (-59.7, 430.39) centre (-56.35, 430.39) ccw
  line L301 (-53, 430.39) -> (-53, 387.09)
  arc A291 (-59.7, 387.09) -> (-53, 387.09) centre (-56.35, 387.09) ccw
  line L302 (-71.9, 387.09) -> (-71.9, 430.39)
  arc A292 (-65.2, 430.39) -> (-71.9, 430.39) centre (-68.55, 430.39) ccw
  line L303 (-65.2, 430.39) -> (-65.2, 387.09)
  arc A293 (-71.9, 387.09) -> (-65.2, 387.09) centre (-68.55, 387.09) ccw
  line L304 (-84.1, 387.09) -> (-84.1, 430.39)
  arc A294 (-77.4, 430.39) -> (-84.1, 430.39) centre (-80.75, 430.39) ccw
  line L305 (-77.4, 430.39) -> (-77.4, 387.09)
  arc A295 (-84.1, 387.09) -> (-77.4, 387.09) centre (-80.75, 387.09) ccw
  line L306 (-96.3, 387.09) -> (-96.3, 430.39)
  arc A296 (-89.6, 430.39) -> (-96.3, 430.39) centre (-92.95, 430.39) ccw
  line L307 (-89.6, 430.39) -> (-89.6, 387.09)
  arc A297 (-96.3, 387.09) -> (-89.6, 387.09) centre (-92.95, 387.09) ccw
  line L308 (-108.5, 387.09) -> (-108.5, 430.39)
  arc A298 (-101.8, 430.39) -> (-108.5, 430.39) centre (-105.15, 430.39) ccw
  line L309 (-101.8, 430.39) -> (-101.8, 387.09)
  arc A299 (-108.5, 387.09) -> (-101.8, 387.09) centre (-105.15, 387.09) ccw
  line L310 (-120.7, 387.09) -> (-120.7, 430.39)
  arc A300 (-114, 430.39) -> (-120.7, 430.39) centre (-117.35, 430.39) ccw
  line L311 (-114, 430.39) -> (-114, 387.09)
  arc A301 (-120.7, 387.09) -> (-114, 387.09) centre (-117.35, 387.09) ccw
  line L312 (-132.9, 387.09) -> (-132.9, 430.39)
  arc A302 (-126.2, 430.39) -> (-132.9, 430.39) centre (-129.55, 430.39) ccw
  line L313 (-126.2, 430.39) -> (-126.2, 387.09)
  arc A303 (-132.9, 387.09) -> (-126.2, 387.09) centre (-129.55, 387.09) ccw
  line L314 (-145.1, 387.09) -> (-145.1, 430.39)
  arc A304 (-138.4, 430.39) -> (-145.1, 430.39) centre (-141.75, 430.39) ccw
  line L315 (-138.4, 430.39) -> (-138.4, 387.09)
  arc A305 (-145.1, 387.09) -> (-138.4, 387.09) centre (-141.75, 387.09) ccw
  line L316 (-157.3, 387.09) -> (-157.3, 430.39)
  arc A306 (-150.6, 430.39) -> (-157.3, 430.39) centre (-153.95, 430.39) ccw
  line L317 (-150.6, 430.39) -> (-150.6, 387.09)
  arc A307 (-157.3, 387.09) -> (-150.6, 387.09) centre (-153.95, 387.09) ccw
  line L318 (-169.5, 387.09) -> (-169.5, 430.39)
  arc A308 (-162.8, 430.39) -> (-169.5, 430.39) centre (-166.15, 430.39) ccw
  line L319 (-162.8, 430.39) -> (-162.8, 387.09)
  arc A309 (-169.5, 387.09) -> (-162.8, 387.09) centre (-166.15, 387.09) ccw
  line L320 (-181.7, 387.09) -> (-181.7, 430.39)
  arc A310 (-175, 430.39) -> (-181.7, 430.39) centre (-178.35, 430.39) ccw
  line L321 (-175, 430.39) -> (-175, 387.09)
  arc A311 (-181.7, 387.09) -> (-175, 387.09) centre (-178.35, 387.09) ccw
  line L322 (-193.9, 387.09) -> (-193.9, 430.39)
  arc A312 (-187.2, 430.39) -> (-193.9, 430.39) centre (-190.55, 430.39) ccw
  line L323 (-187.2, 430.39) -> (-187.2, 387.09)
  arc A313 (-193.9, 387.09) -> (-187.2, 387.09) centre (-190.55, 387.09) ccw
  line L324 (-206.1, 387.09) -> (-206.1, 430.39)
  arc A314 (-199.4, 430.39) -> (-206.1, 430.39) centre (-202.75, 430.39) ccw
  line L325 (-199.4, 430.39) -> (-199.4, 387.09)
  arc A315 (-206.1, 387.09) -> (-199.4, 387.09) centre (-202.75, 387.09) ccw
  line L326 (-218.3, 387.09) -> (-218.3, 430.39)
  arc A316 (-211.6, 430.39) -> (-218.3, 430.39) centre (-214.95, 430.39) ccw
  line L327 (-211.6, 430.39) -> (-211.6, 387.09)
  arc A317 (-218.3, 387.09) -> (-211.6, 387.09) centre (-214.95, 387.09) ccw
  line L328 (-230.5, 387.09) -> (-230.5, 430.39)
  arc A318 (-223.8, 430.39) -> (-230.5, 430.39) centre (-227.15, 430.39) ccw
  line L329 (-223.8, 430.39) -> (-223.8, 387.09)
  arc A319 (-230.5, 387.09) -> (-223.8, 387.09) centre (-227.15, 387.09) ccw
  line L330 (-242.7, 387.09) -> (-242.7, 430.39)
  arc A320 (-236, 430.39) -> (-242.7, 430.39) centre (-239.35, 430.39) ccw
  line L331 (-236, 430.39) -> (-236, 387.09)
  arc A321 (-242.7, 387.09) -> (-236, 387.09) centre (-239.35, 387.09) ccw
  line L332 (-254.9, 387.09) -> (-254.9, 430.39)
  arc A322 (-248.2, 430.39) -> (-254.9, 430.39) centre (-251.55, 430.39) ccw
  line L333 (-248.2, 430.39) -> (-248.2, 387.09)
  arc A323 (-254.9, 387.09) -> (-248.2, 387.09) centre (-251.55, 387.09) ccw
  line L334 (-267.1, 387.09) -> (-267.1, 430.39)
  arc A324 (-260.4, 430.39) -> (-267.1, 430.39) centre (-263.75, 430.39) ccw
  line L335 (-260.4, 430.39) -> (-260.4, 387.09)
  arc A325 (-267.1, 387.09) -> (-260.4, 387.09) centre (-263.75, 387.09) ccw
  line L336 (-279.3, 387.09) -> (-279.3, 430.39)
  arc A326 (-272.6, 430.39) -> (-279.3, 430.39) centre (-275.95, 430.39) ccw
  line L337 (-272.6, 430.39) -> (-272.6, 387.09)
  arc A327 (-279.3, 387.09) -> (-272.6, 387.09) centre (-275.95, 387.09) ccw
  line L338 (-291.5, 387.09) -> (-291.5, 430.39)
  arc A328 (-284.8, 430.39) -> (-291.5, 430.39) centre (-288.15, 430.39) ccw
  line L339 (-284.8, 430.39) -> (-284.8, 387.09)
  arc A329 (-291.5, 387.09) -> (-284.8, 387.09) centre (-288.15, 387.09) ccw
  line L340 (-303.7, 387.09) -> (-303.7, 430.39)
  arc A330 (-297, 430.39) -> (-303.7, 430.39) centre (-300.35, 430.39) ccw
  line L341 (-297, 430.39) -> (-297, 387.09)
  arc A331 (-303.7, 387.09) -> (-297, 387.09) centre (-300.35, 387.09) ccw
  line L342 (-315.9, 387.09) -> (-315.9, 430.39)
  arc A332 (-309.2, 430.39) -> (-315.9, 430.39) centre (-312.55, 430.39) ccw
  line L343 (-309.2, 430.39) -> (-309.2, 387.09)
  arc A333 (-315.9, 387.09) -> (-309.2, 387.09) centre (-312.55, 387.09) ccw
  line L344 (-328.1, 387.09) -> (-328.1, 430.39)
  arc A334 (-321.4, 430.39) -> (-328.1, 430.39) centre (-324.75, 430.39) ccw
  line L345 (-321.4, 430.39) -> (-321.4, 387.09)
  arc A335 (-328.1, 387.09) -> (-321.4, 387.09) centre (-324.75, 387.09) ccw
  line L346 (-340.3, 387.09) -> (-340.3, 430.39)
  arc A336 (-333.6, 430.39) -> (-340.3, 430.39) centre (-336.95, 430.39) ccw
  line L347 (-333.6, 430.39) -> (-333.6, 387.09)
  arc A337 (-340.3, 387.09) -> (-333.6, 387.09) centre (-336.95, 387.09) ccw
  line L348 (-352.5, 387.09) -> (-352.5, 430.39)
  arc A338 (-345.8, 430.39) -> (-352.5, 430.39) centre (-349.15, 430.39) ccw
  line L349 (-345.8, 430.39) -> (-345.8, 387.09)
  arc A339 (-352.5, 387.09) -> (-345.8, 387.09) centre (-349.15, 387.09) ccw
  line L350 (-364.7, 387.09) -> (-364.7, 430.39)
  arc A340 (-358, 430.39) -> (-364.7, 430.39) centre (-361.35, 430.39) ccw
  line L351 (-358, 430.39) -> (-358, 387.09)
  arc A341 (-364.7, 387.09) -> (-358, 387.09) centre (-361.35, 387.09) ccw
  line L352 (-35.3, 447.09) -> (-35.3, 490.39)
  arc A342 (-28.6, 490.39) -> (-35.3, 490.39) centre (-31.95, 490.39) ccw
  line L353 (-28.6, 490.39) -> (-28.6, 447.09)
  arc A343 (-35.3, 447.09) -> (-28.6, 447.09) centre (-31.95, 447.09) ccw
  line L354 (-47.5, 447.09) -> (-47.5, 490.39)
  arc A344 (-40.8, 490.39) -> (-47.5, 490.39) centre (-44.15, 490.39) ccw
  line L355 (-40.8, 490.39) -> (-40.8, 447.09)
  arc A345 (-47.5, 447.09) -> (-40.8, 447.09) centre (-44.15, 447.09) ccw
  line L356 (-59.7, 447.09) -> (-59.7, 490.39)
  arc A346 (-53, 490.39) -> (-59.7, 490.39) centre (-56.35, 490.39) ccw
  line L357 (-53, 490.39) -> (-53, 447.09)
  arc A347 (-59.7, 447.09) -> (-53, 447.09) centre (-56.35, 447.09) ccw
  line L358 (-71.9, 447.09) -> (-71.9, 490.39)
  arc A348 (-65.2, 490.39) -> (-71.9, 490.39) centre (-68.55, 490.39) ccw
  line L359 (-65.2, 490.39) -> (-65.2, 447.09)
  arc A349 (-71.9, 447.09) -> (-65.2, 447.09) centre (-68.55, 447.09) ccw
  line L360 (-84.1, 447.09) -> (-84.1, 490.39)
  arc A350 (-77.4, 490.39) -> (-84.1, 490.39) centre (-80.75, 490.39) ccw
  line L361 (-77.4, 490.39) -> (-77.4, 447.09)
  arc A351 (-84.1, 447.09) -> (-77.4, 447.09) centre (-80.75, 447.09) ccw
  line L362 (-96.3, 447.09) -> (-96.3, 490.39)
  arc A352 (-89.6, 490.39) -> (-96.3, 490.39) centre (-92.95, 490.39) ccw
  line L363 (-89.6, 490.39) -> (-89.6, 447.09)
  arc A353 (-96.3, 447.09) -> (-89.6, 447.09) centre (-92.95, 447.09) ccw
  line L364 (-108.5, 447.09) -> (-108.5, 490.39)
  arc A354 (-101.8, 490.39) -> (-108.5, 490.39) centre (-105.15, 490.39) ccw
  line L365 (-101.8, 490.39) -> (-101.8, 447.09)
  arc A355 (-108.5, 447.09) -> (-101.8, 447.09) centre (-105.15, 447.09) ccw
  line L366 (-120.7, 447.09) -> (-120.7, 490.39)
  arc A356 (-114, 490.39) -> (-120.7, 490.39) centre (-117.35, 490.39) ccw
  line L367 (-114, 490.39) -> (-114, 447.09)
  arc A357 (-120.7, 447.09) -> (-114, 447.09) centre (-117.35, 447.09) ccw
  line L368 (-132.9, 447.09) -> (-132.9, 490.39)
  arc A358 (-126.2, 490.39) -> (-132.9, 490.39) centre (-129.55, 490.39) ccw
  line L369 (-126.2, 490.39) -> (-126.2, 447.09)
  arc A359 (-132.9, 447.09) -> (-126.2, 447.09) centre (-129.55, 447.09) ccw
  line L370 (-145.1, 447.09) -> (-145.1, 490.39)
  arc A360 (-138.4, 490.39) -> (-145.1, 490.39) centre (-141.75, 490.39) ccw
  line L371 (-138.4, 490.39) -> (-138.4, 447.09)
  arc A361 (-145.1, 447.09) -> (-138.4, 447.09) centre (-141.75, 447.09) ccw
  line L372 (-157.3, 447.09) -> (-157.3, 490.39)
  arc A362 (-150.6, 490.39) -> (-157.3, 490.39) centre (-153.95, 490.39) ccw
  line L373 (-150.6, 490.39) -> (-150.6, 447.09)
  arc A363 (-157.3, 447.09) -> (-150.6, 447.09) centre (-153.95, 447.09) ccw
  line L374 (-169.5, 447.09) -> (-169.5, 490.39)
  arc A364 (-162.8, 490.39) -> (-169.5, 490.39) centre (-166.15, 490.39) ccw
  line L375 (-162.8, 490.39) -> (-162.8, 447.09)
  arc A365 (-169.5, 447.09) -> (-162.8, 447.09) centre (-166.15, 447.09) ccw
  line L376 (-181.7, 447.09) -> (-181.7, 490.39)
  arc A366 (-175, 490.39) -> (-181.7, 490.39) centre (-178.35, 490.39) ccw
  line L377 (-175, 490.39) -> (-175, 447.09)
  arc A367 (-181.7, 447.09) -> (-175, 447.09) centre (-178.35, 447.09) ccw
  line L378 (-193.9, 447.09) -> (-193.9, 490.39)
  arc A368 (-187.2, 490.39) -> (-193.9, 490.39) centre (-190.55, 490.39) ccw
  line L379 (-187.2, 490.39) -> (-187.2, 447.09)
  arc A369 (-193.9, 447.09) -> (-187.2, 447.09) centre (-190.55, 447.09) ccw
  line L380 (-206.1, 447.09) -> (-206.1, 490.39)
  arc A370 (-199.4, 490.39) -> (-206.1, 490.39) centre (-202.75, 490.39) ccw
  line L381 (-199.4, 490.39) -> (-199.4, 447.09)
  arc A371 (-206.1, 447.09) -> (-199.4, 447.09) centre (-202.75, 447.09) ccw
  line L382 (-218.3, 447.09) -> (-218.3, 490.39)
  arc A372 (-211.6, 490.39) -> (-218.3, 490.39) centre (-214.95, 490.39) ccw
  line L383 (-211.6, 490.39) -> (-211.6, 447.09)
  arc A373 (-218.3, 447.09) -> (-211.6, 447.09) centre (-214.95, 447.09) ccw
  line L384 (-230.5, 447.09) -> (-230.5, 490.39)
  arc A374 (-223.8, 490.39) -> (-230.5, 490.39) centre (-227.15, 490.39) ccw
  line L385 (-223.8, 490.39) -> (-223.8, 447.09)
  arc A375 (-230.5, 447.09) -> (-223.8, 447.09) centre (-227.15, 447.09) ccw
  line L386 (-242.7, 447.09) -> (-242.7, 490.39)
  arc A376 (-236, 490.39) -> (-242.7, 490.39) centre (-239.35, 490.39) ccw
  line L387 (-236, 490.39) -> (-236, 447.09)
  arc A377 (-242.7, 447.09) -> (-236, 447.09) centre (-239.35, 447.09) ccw